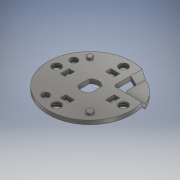
# Autodesk Inventor part: Część1
Saved by Autodesk Inventor 2017 SP1 (Build 210196100, 196)
## iProperties
Created: 2021-01-12
Part Number: Część1
Material: Stal, galwanizowana
Document SubType Name: Modeling
Designer: Napoleon
Mass: 15.8681 g
Surface Area: 26.381 cm^2
Volume: 2.02142 cm^3
Density: 7.85 g/cm^3
Appearance: Galwanizowana
Author: Napoleon
Autodesk Inventor part; units mm, degrees
ref_plane "YZ Plane" through (0, 0, 0) normal (1, 0, 0) x (0, 1, 0)
ref_plane "XZ Plane" through (0, 0, 0) normal (0, 1, 0) x (-1, 0, 0)
sketch "Szkic1" plane through (0, 0, 0) normal (0, 0, 1) x (1, 0, 0)
  arc A0 (5.4476, 18.6976) -> (18.6976, 5.4476) centre (0, 0) ccw
  line L0 (-11.75, 2.05) -> (-9.25, 2.05)
  line L1 (-9.25, 2.05) -> (-9.25, -2.05)
  line L2 (-9.25, -2.05) -> (-11.75, -2.05)
  line L3 (-11.75, -2.05) -> (-11.75, 2.05)
  line L4 (-2.05, -11.75) -> (-2.05, -9.25)
  line L5 (-2.05, -9.25) -> (2.05, -9.25)
  line L6 (2.05, -9.25) -> (2.05, -11.75)
  line L7 (2.05, -11.75) -> (-2.05, -11.75)
  line L8 (11.75, -2.05) -> (9.25, -2.05)
  line L9 (9.25, -2.05) -> (9.25, 2.05)
  line L10 (9.25, 2.05) -> (11.75, 2.05)
  line L11 (11.75, 2.05) -> (11.75, -2.05)
  line L12 (2.05, 11.75) -> (2.05, 9.25)
  line L13 (2.05, 9.25) -> (-2.05, 9.25)
  line L14 (-2.05, 9.25) -> (-2.05, 11.75)
  line L15 (-2.05, 11.75) -> (2.05, 11.75)
  line L16 (18.6976, 5.4476) -> (5.4476, 5.4476)
  line L17 (5.4476, 5.4476) -> (5.4476, 18.6976)
  circle A1 centre (0, 15.5) radius 2
  line L18 (-3, -2.6458) -> (-3, 2.6458)
  line L19 (3, 2.6458) -> (3, -2.6458)
  arc A2 (-3, -2.6458) -> (3, -2.6458) centre (0, 0) ccw
  arc A3 (3, 2.6458) -> (-3, 2.6458) centre (0, 0) ccw
  circle A4 centre (-15.5, 0) radius 2
  circle A5 centre (0, -15.5) radius 2
  circle A6 centre (15.5, 0) radius 2
  circle A7 centre (-14.0478, 6.5506) radius 1.7
  line L20 (-15.5, 0) -> (-12.5, 0) construction
  circle A8 centre (-6.5506, -14.0478) radius 1.7
  dimension "d0" = 38.95
  dimension "d5" = 2.5
  dimension "d6" = 4.1
  dimension "d9" = 360
  dimension "d12" = 13.25
  dimension "d14" = 4
  dimension "d19" = 360
  constraints: 42 end point, 9 centre point, 6 point on circle, 3 horizontal, 3 parallel, 2 perpendicular, 1 coincident, 42 other
  measures "d0" diameter of A0
  measures "d5" distance of L1.end L2.end
  measures "d6" distance of L0.end L1.end
  measures "d12" distance of L16.end L17.end
  measures "d14" diameter of A1
extrude "Wyciągnięcie proste1" add sketch "Szkic1" against normal blind 2
fillet "Zaokrąglenie1" radius 0.25 1 edges at (-13.7709, -13.7709, -2)
thread "Gwint1" size "M4x0.7" class "6H" standard "ANSI Metric M Profile" full length
thread "Gwint2" size "M4x0.7" class "6H" standard "ANSI Metric M Profile" full length
thread "Gwint3" size "M4x0.7" class "6H" standard "ANSI Metric M Profile" full length
thread "Gwint4" size "M4x0.7" class "6H" standard "ANSI Metric M Profile" full length
fillet "Zaokrąglenie2" radius 1 1 edges at (5.4476, 5.4476, -1)
sketch "Szkic2" plane through (0, 0, 0) normal (0, 0, 1) x (1, 0, 0)
  circle A0 centre (10.9602, -10.9602) radius 1.55
  circle A1 centre (-10.9602, 10.9602) radius 1.275
  dimension "d42" = 3.1
  dimension "d69" = 2.55
  constraints: 2 centre point
  measures "d42" diameter of A0
  measures "d69" diameter of A1
extrude "Wyciągnięcie proste2" add sketch "Szkic2" along normal blind 1.15
fillet "Zaokrąglenie3" radius 0.2 1 edges at (9.4102, -10.9602, 1.15)
ref_plane "Płaszczyzna konstrukcyjna1" through (0, 0, -4.5) normal (0, 0, -1) x (-1, 0, 0)
sketch "Szkic3" plane through (0, 0, -4.5) normal (0, 0, -1) x (-1, 0, 0)
  arc A0 (-7.973, 17.7681) -> (-17.7795, 7.9476) centre (0, 0) ccw
  line L0 (-7.973, 8.9476) -> (-7.973, 17.7681)
  line L1 (-8.973, 7.9476) -> (-17.7795, 7.9476)
  line L2 (-7.973, 8.9476) -> (-8.973, 7.9476)
  point P0 (-7.973, 7.9476)
  dimension "d53" = 1
  dimension "d54" = 45
  constraints: 6 end point, 2 point on circle, 2 point on line, 1 centre point, 1 coincident, 1 horizontal, 1 vertical
  measures "d53" distance of L0.start point (-7.973, 7.948)
  measures "d54" angle of L0 L2
extrude "Wyciągnięcie proste3" add sketch "Szkic3" against normal blind 2
fillet "Zaokrąglenie4" radius 0.25 1 edges at (13.7807, 13.7611, -4.5)
sketch "Szkic4" plane through (5.4476, 18.6976, 0) normal (1, 0, 0) x (0, 0, -1)
  spline S0 degree 3 poles (1.75, 0) (1.7804, 0) (1.8162, -0.0073) (1.8729, -0.0314) (1.9036, -0.0525) (1.9476, -0.0976) (1.9684, -0.1298) (1.9926, -0.1895) (2, -0.2279) (2, -0.2605) knots 0.151278 0.151278 0.151278 0.151278 0.160412 0.160412 0.16974 0.16974 0.179309 0.179309 0.189088 0.189088 0.189088 0.189088
  line L0 (0, 0) -> (1.75, 0)
  line L1 (0, 0) -> (0, -5.2605)
  line L2 (2, -0.2605) -> (2, -5.2605)
  line L3 (2, -5.2605) -> (0, -5.2605)
  dimension "d58" = 5
  constraints: 8 end point, 1 horizontal, 1 vertical, 2 other
  measures "d58" distance of L2.start L2.end
sketch "Szkic5" plane through (7.973, 8.9476, -2.5) normal (-1, 0, 0) x (0, 0, 1)
  spline S0 degree 3 poles (-2, 8.5462) (-2, 8.5811) (-1.9924, 8.6223) (-1.9675, 8.6857) (-1.9464, 8.7196) (-1.9019, 8.7666) (-1.8713, 8.7885) (-1.8151, 8.8131) (-1.7799, 8.8206) (-1.75, 8.8206) knots 0.116657 0.116657 0.116657 0.116657 0.12713 0.12713 0.137107 0.137107 0.146527 0.146527 0.15551 0.15551 0.15551 0.15551
  line L0 (-1.75, 8.8206) -> (0, 8.8206)
  line L1 (0, 4.5524) -> (-2, 4.5524)
  line L2 (-2, 4.5524) -> (-2, 8.5462)
  line L3 (0, 8.8206) -> (0, 4.5524)
  point P0 (2.5, -8.9476)
  constraints: 8 end point, 1 horizontal, 1 vertical, 2 other
loft "Wyciągnięcie złożone1" add profiles "Szkic5", "Szkic4"
sketch "Szkic6" plane through (18.6976, 5.4476, 0) normal (0, 1, 0) x (1, 0, 0)
  line L0 (0, 0) -> (0, 1.75)
  spline S0 degree 3 poles (-0.2605, 2) (-0.2279, 2) (-0.1895, 1.9926) (-0.1298, 1.9684) (-0.0976, 1.9476) (-0.0525, 1.9036) (-0.0314, 1.8729) (-0.0073, 1.8162) (0, 1.7804) (0, 1.75) knots 0.113468 0.113468 0.113468 0.113468 0.123246 0.123246 0.132815 0.132815 0.142143 0.142143 0.151278 0.151278 0.151278 0.151278
  line L1 (0, 0) -> (-5, 0)
  line L2 (-5, 0) -> (-5, 2)
  line L3 (-5, 2) -> (-0.2605, 2)
  point P0 (-18.6976, 0)
  point P1 (-13.25, 0)
  dimension "d63" = 5
  constraints: 8 end point, 2 perpendicular, 2 other
  measures "d63" distance of L0.start L1.end
sketch "Szkic7" plane through (8.973, 7.9476, -2.5) normal (0, -1, 0) x (1, 0, 0)
  spline S0 degree 3 poles (8.8065, -1.75) (8.8065, -1.78) (8.7991, -1.8151) (8.7745, -1.8713) (8.7526, -1.902) (8.7056, -1.9464) (8.6718, -1.9675) (8.6084, -1.9924) (8.5672, -2) (8.5323, -2) knots 0.155455 0.155455 0.155455 0.155455 0.164441 0.164441 0.17386 0.17386 0.183832 0.183832 0.194295 0.194295 0.194295 0.194295
  line L0 (8.8065, -1.75) -> (8.8065, 0)
  line L1 (4.527, 0) -> (4.527, -2)
  line L2 (8.5323, -2) -> (4.527, -2)
  line L3 (8.8065, 0) -> (4.527, 0)
  point P0 (-8.973, 2.5)
  constraints: 8 end point, 1 vertical, 2 other
loft "Wyciągnięcie złożone2" add profiles "Szkic7", "Szkic6"
fillet "Zaokrąglenie5" radius 0.2 1 edges at (-12.2352, 10.9602, 1.15)
